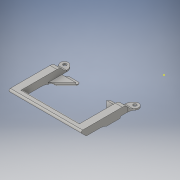
# Autodesk Inventor part: battery_clip
Saved by Autodesk Inventor 2016 (Build 200138000, 138)
## iProperties
Created: 2016-03-06
Part Number: battery_clip
Material: Generic
Document SubType Name: Modeling
Designer: dimas
Density: 1 g/cm^3
Appearance: Default
Author: dimas
Autodesk Inventor part; units mm, degrees
ref_plane "YZ Plane" through (0, 0, 0) normal (1, 0, 0) x (0, 1, 0)
ref_plane "XZ Plane" through (0, 0, 0) normal (0, 1, 0) x (-1, 0, 0)
ref_plane "XY Plane" through (0, 0, 0) normal (0, 0, 1) x (1, 0, 0)
sketch "Sketch1" plane through (0, 0, 0) normal (0, 1, 0) x (-1, 0, 0)
  line L0 (0, 0) -> (0, 76.2)
  line L1 (0, 76.2) -> (53.34, 76.2)
  line L2 (53.34, 76.2) -> (53.34, 0)
  line L3 (53.34, 0) -> (59.69, 0)
  line L4 (59.69, 0) -> (59.69, 82.55)
  line L5 (0, 0) -> (-6.35, 0)
  line L6 (-6.35, 0) -> (-6.35, 82.55)
  line L7 (-6.35, 82.55) -> (59.69, 82.55)
  dimension "d0" = 76.2
  dimension "d1" = 53.34
  dimension "d2" = 6.35
  dimension "d3" = 82.55
  dimension "d4" = 6.35
  dimension "d5" = 82.55
  constraints: 16 end point, 4 perpendicular, 3 horizontal, 1 vertical
  measures "d0" distance of L0.start L0.end
  measures "d1" distance of L0.end L1.end
  measures "d2" distance of L2.end L3.end
  measures "d3" distance of L3.end L4.end
  measures "d4" distance of L0.start L5.end
  measures "d5" distance of L5.end L6.end
extrude "Extrusion1" add sketch "Sketch1" along normal blind 6.35
sketch "Sketch2" plane through (0, 0, 0) normal (0, -1, 0) x (1, 0, 0)
  line L0 (6.35, 0) -> (0, 0) projected
  line L1 (6.35, 0) -> (6.35, 40.005)
  line L2 (6.35, 82.55) -> (6.35, 0) projected
  line L3 (-59.69, 0) -> (-59.69, 82.55) projected
  line L4 (6.35, 40.005) -> (-59.69, 40.005)
  line L5 (-59.69, 40.005) -> (-59.69, 46.355)
  line L6 (-59.69, 46.355) -> (6.35, 46.355)
  line L7 (6.35, 46.355) -> (6.35, 40.005)
  dimension "d17" = 40.005
  dimension "d18" = 6.35
  constraints: 10 end point, 2 parallel, 2 point on line, 1 horizontal, 1 perpendicular
  measures "d17" distance of L0.start L1.end
  measures "d18" distance of L4.end L5.end
extrude "Extrusion2" add sketch "Sketch2" along normal blind 1.524
sketch "Sketch3" plane through (0, -1.524, 0) normal (0, -1, 0) x (1, 0, 0)
  line L0 (-59.69, 40.005) -> (6.35, 40.005) projected
  line L1 (6.35, 40.005) -> (0, 40.005)
  line L2 (6.35, 46.355) -> (-59.69, 46.355) projected
  line L3 (0, 40.005) -> (6.35, 46.355)
  line L4 (6.35, 46.355) -> (6.35, 40.005)
  line L5 (-59.69, 40.005) -> (-59.69, 46.355)
  line L6 (-59.69, 40.005) -> (-53.34, 40.005)
  line L7 (-53.34, 40.005) -> (-59.69, 46.355)
  line L8 (6.35, 40.005) -> (6.35, 46.355)
  line L9 (6.35, 82.55) -> (6.35, 0) projected
  line L10 (6.35, 46.355) -> (0, 40.005)
  line L11 (0, 40.005) -> (6.35, 40.005)
  point P0 (0, 0)
  dimension "d21" = 6.35
  dimension "d22" = 6.35
  constraints: 18 end point, 2 collinear, 2 point on line, 1 perpendicular, 1 vertical
  measures "d21" distance of L0.end L1.end
  measures "d22" distance of L0.start L6.end
extrude "Extrusion3" cut sketch "Sketch3" against normal blind 1.524 contours L5 L7 L0 | L3 L4 L0
sketch "Sketch4" plane through (0, 0, 0) normal (0, -1, 0) x (1, 0, 0)
  line L0 (-59.69, 46.355) -> (-53.34, 40.005) projected
  line L1 (-53.34, 40.005) -> (-53.34, 36.83)
  line L2 (-53.34, 40.005) -> (-53.34, 0) projected
  line L3 (-53.34, 36.83) -> (-64.6008, 36.83)
  line L4 (-64.6008, 36.83) -> (19.5424, 36.83)
  line L5 (19.5424, 36.83) -> (19.5424, -15.2402)
  line L6 (19.5424, -15.2402) -> (-64.6008, -15.2402)
  line L7 (-64.6008, -15.2402) -> (-64.6008, 36.83)
  point P0 (0, 0)
  dimension "d25" = 3.175
  constraints: 12 end point, 2 parallel, 2 perpendicular, 1 horizontal, 1 point on line
  measures "d25" distance of L0.end L1.end
extrude "Extrusion4" cut sketch "Sketch4" against normal through all
chamfer "Chamfer4" distance 5.08 angle 45 2 edges at (-56.515, 6.35, 36.83) (3.175, 6.35, 36.83)
sketch "Sketch5" plane through (0, -1.524, 0) normal (0, -1, 0) x (1, 0, 0)
  line L0 (6.35, 46.355) -> (-59.69, 46.355) projected
  line L1 (6.35, 46.355) -> (6.35, 59.055)
  line L2 (6.35, 82.55) -> (6.35, 46.355) projected
  line L3 (6.35, 46.355) -> (-6.35, 46.355)
  line L4 (0, 46.355) -> (-53.34, 46.355) projected
  line L5 (-6.35, 46.355) -> (6.35, 59.055)
  line L6 (-59.69, 46.355) -> (-59.69, 59.055)
  line L7 (-59.69, 41.91) -> (-59.69, 82.55) projected
  line L8 (-59.69, 46.355) -> (-46.99, 46.355)
  line L9 (-46.99, 46.355) -> (-59.69, 59.055)
  point P0 (0, 0)
  dimension "d31" = 12.7
  dimension "d32" = 12.7
  dimension "d33" = 12.7
  dimension "d34" = 12.7
  constraints: 12 end point, 4 point on line
  measures "d31" distance of L0.start L1.end
  measures "d32" distance of L0.start L3.end
  measures "d33" distance of L0.end L6.end
  measures "d34" distance of L0.end L8.end
extrude "Extrusion5" add sketch "Sketch5" against normal blind 1.524
chamfer "Chamfer5" distance 5.08 angle 45 1 edges at (-26.67, 0, 82.55)
sketch "Sketch7" plane through (0, 6.35, 0) normal (0, 1, 0) x (1, 0, 0)
  point P0 (0, 0)
fillet "Fillet1" radius 6.35 2 edges at (3.175, 0, 55.88) (-56.515, 0, 55.88)
fillet "Fillet2" radius 6.35 2 edges at (-56.515, 6.35, 41.91) (3.175, 6.35, 41.91)
fillet "Fillet3" radius 1.27 2 edges at (-26.67, 6.35, 82.55) (-26.67, 5.08, 82.55)
fillet "Fillet4" radius 1.27 2 edges at (-26.67, 0, 77.47) (-26.67, 0, 76.2)
fillet "Fillet5" radius 1.27 1 edges at (-26.67, 6.35, 76.2)
sketch "Sketch8" plane through (0, 0, 0) normal (0, -1, 0) x (1, 0, 0)
  line L0 (0, 36.83) -> (0, 40.005) projected
  line L1 (-53.34, 40.005) -> (0, 40.005) projected
  line L2 (0, 36.83) -> (0, 32.004)
  line L3 (0, 36.83) -> (6.35, 36.83) projected
  line L4 (6.35, 27.178) -> (0, 32.004)
  line L5 (6.35, 27.178) -> (10.1923, 32.2336)
  line L6 (10.1923, 32.2336) -> (6.35, 36.83)
  circle A0 centre (5.334, 32.004) radius 1.5
  line L7 (-53.34, 36.83) -> (-59.69, 36.83) projected
  line L8 (-53.34, 36.83) -> (-53.34, 32.004)
  line L9 (-59.69, 27.178) -> (-53.34, 32.004)
  line L10 (-59.69, 27.178) -> (-63.5323, 32.2336)
  line L11 (-63.5323, 32.2336) -> (-59.69, 36.83)
  line L12 (-59.69, 36.83) -> (-53.34, 36.83)
  line L13 (6.35, 36.83) -> (0, 36.83)
  circle A1 centre (-58.674, 32.004) radius 1.5
  point P0 (0, 0)
  dimension "d45" = 8.001
  dimension "d48" = 9.652
  dimension "d49" = 6.35
  dimension "d50" = 3
  dimension "d51" = 9.652
  dimension "d52" = 6.35
  dimension "d53" = 3
  constraints: 20 end point, 2 centre point, 2 collinear, 2 perpendicular, 1 vertical
  measures "d45" distance of L0.end L2.end
  measures "d48" distance of L3.end L4.start
  measures "d49" distance of L4.start L5.end
  measures "d50" diameter of A0
  measures "d51" distance of L7.end L9.start
  measures "d52" distance of L9.start L10.end
  measures "d53" diameter of A1
extrude "Extrusion6" add sketch "Sketch8" against normal blind 1.27
fillet "Fillet6" radius 2.54 2 edges at (3.175, 1.27, 36.83) (-56.515, 1.27, 36.83)
fillet "Fillet7" radius 3.556 2 edges at (10.1923, 0.635, 32.2336) (6.35, 0.635, 27.178)
fillet "Fillet8" radius 8.128 1 edges at (6.35, 0.7491, 36.83)
fillet "Fillet9" radius 7.62 1 edges at (0, 0.635, 32.004)
fillet "Fillet10" radius 3.556 2 edges at (-59.69, 0.635, 27.178) (-63.5323, 0.635, 32.2336)
fillet "Fillet11" radius 8.382 1 edges at (-59.69, 0.7491, 36.83)
fillet "Fillet12" radius 7.62 1 edges at (-53.34, 0.635, 32.004)
sketch "Sketch9" plane through (0, -1.524, 0) normal (0, -1, 0) x (1, 0, 0)
  line L0 (-6.35, 46.355) -> (-46.99, 46.355) projected
  line L1 (-6.35, 46.355) -> (-12.7, 40.005)
  line L2 (-53.34, 40.005) -> (0, 40.005) projected
  line L3 (0, 52.705) -> (-6.35, 46.355) projected
  line L4 (-46.99, 46.355) -> (-40.64, 40.005)
  line L5 (-53.34, 52.705) -> (-46.99, 46.355) projected
  line L6 (-40.64, 40.005) -> (-12.7, 40.005)
  line L7 (-6.35, 46.355) -> (-46.99, 46.355)
  point P0 (0, 0)
  constraints: 8 end point, 3 collinear, 2 point on line, 1 parallel
extrude "Extrusion7" cut sketch "Sketch9" against normal through all
sketch "Sketch10" plane through (0, -1.524, 0) normal (0, -1, 0) x (1, 0, 0)
  line L0 (0, 40.005) -> (6.35, 46.355) projected
  line L1 (3.175, 43.18) -> (-5.8053, 34.1997)
  line L2 (3.175, 43.18) -> (-3.175, 49.53)
  line L3 (-12.7, 40.005) -> (0, 52.705) projected
  line L4 (-3.175, 49.53) -> (-18.5053, 34.1997)
  line L5 (-18.5053, 34.1997) -> (-5.8053, 34.1997)
  line L6 (-59.69, 46.355) -> (-53.34, 40.005) projected
  line L7 (-56.515, 43.18) -> (-47.5347, 34.1997)
  line L8 (-56.515, 43.18) -> (-50.165, 49.53)
  line L9 (-50.165, 49.53) -> (-34.8347, 34.1997)
  line L10 (-34.8347, 34.1997) -> (-47.5347, 34.1997)
  point P0 (0, 0)
  dimension "d65" = 12.7
  dimension "d66" = 12.7
  constraints: 16 end point, 2 collinear, 2 horizontal, 2 midpoint, 2 point on line, 1 perpendicular
  measures "d65" distance of L1.start L1.end
  measures "d66" distance of L7.start L7.end
extrude "Extrusion8" add sketch "Sketch10" along normal blind 1.524
chamfer "Chamfer6" distance 1.524 angle 45 2 edges at (0, -1.524, 46.355) (-53.34, -1.524, 46.355)
fillet "Fillet13" radius 2.54 1 edges at (1.0776, -1.524, 47.4326)
fillet "Fillet14" radius 2.54 1 edges at (-54.4176, -1.524, 47.4326)
fillet "Fillet15" radius 2.54 4 edges at (-50.165, -3.048, 49.53) (-53.34, -3.0479, 46.355) (-53.34, -3.048, 46.355) (-56.515, -3.048, 43.18)
fillet "Fillet16" radius 2.54 4 edges at (3.175, -3.048, 43.18) (-3.175, -3.048, 49.53) (0, -3.0479, 46.355) (0, -3.048, 46.355)
sketch "Sketch11" plane through (-34.8347, -1.524, 34.1997) normal (0, 0, -1) x (-1, 0, 0)
  line L0 (18.5053, 7.874) -> (-34.8347, 7.874) projected
  line L1 (-34.8347, 7.874) -> (18.5053, 7.874)
  line L2 (18.5053, 7.874) -> (18.5053, -5.1086)
  line L3 (18.5053, -5.1086) -> (-34.8347, -5.1086)
  line L4 (-34.8347, -5.1086) -> (-34.8347, 7.874)
  point P0 (-34.8347, 1.524)
  constraints: 8 end point, 2 parallel, 1 horizontal, 1 perpendicular
extrude "Extrusion9" cut sketch "Sketch11" against normal blind 2.54
fillet "Fillet17" radius 1.778 2 edges at (-15.9653, -2.286, 36.7397) (-37.3747, -2.286, 36.7397)
fillet "Fillet18" radius 1.27 14 edges at (-7.469, -3.048, 36.7397) (-13.3154, -3.048, 37.8373) (-8.4245, -3.048, 44.2805) (-3.2317, -2.8547, 49.4733) (-2.6363, -2.286, 50.0687) (-2.0408, -1.7173, 50.6642) (-0.6767, -1.524, 52.0283) (-50.1083, -2.8547, 49.4733) (-50.7037, -2.286, 50.0687) (-51.2992, -1.7173, 50.6642) (-52.6633, -1.524, 52.0283) (-40.0246, -3.048, 37.8373) (-45.871, -3.048, 36.7397) (-44.9155, -3.048, 44.2805)
body "Solid1"
